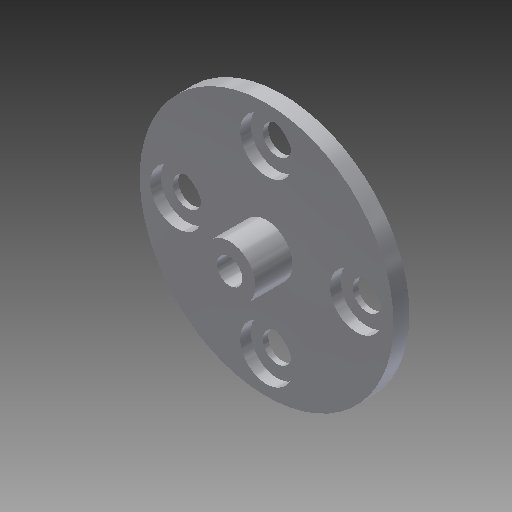
# Autodesk Inventor part: 足首_独立ピッチ_1_2
Saved by Autodesk Inventor 2018 (Build 220112000, 112)
## iProperties
Created: 2016-05-04
Part Number: 足首_独立ピッチ_1_2
Material: アルミニウム 2014-T4
Document SubType Name: Modeling
Designer: hiroaki
Density: 2.8 g/cm^3
Appearance: サテン
Mass: 1.76953 g
Surface Area: 11.344 cm^2
Volume: 0.631975 cm^3
Author: hiroaki
Autodesk Inventor part; units mm, degrees
ref_plane "YZ Plane" through (0, 0, 0) normal (1, 0, 0) x (0, 1, 0)
ref_plane "XZ Plane" through (0, 0, 0) normal (0, 1, 0) x (-1, 0, 0)
ref_plane "XY Plane" through (0, 0, 0) normal (0, 0, 1) x (1, 0, 0)
sketch "スケッチ1" plane through (0, 0, 0) normal (0, 0, 1) x (1, 0, 0)
  circle A0 centre (0, 0) radius 12
  circle A1 centre (0, 8.5) radius 1.35
  circle A2 centre (0, 0) radius 1.2
  circle A3 centre (-8.5, 0) radius 1.35
  circle A4 centre (0, -8.5) radius 1.35
  circle A5 centre (8.5, 0) radius 1.35
  dimension "d0" = 2.7
  dimension "d1" = 8.5
  dimension "d2" = 24
  dimension "d3" = 2.4
  dimension "d6" = 360
  constraints: 6 centre point, 2 coincident, 1 vertical alignment, 9 other
  measures "d0" diameter of A1
  measures "d1" distance of point (0, 0) A1.centre
  measures "d2" diameter of A0
  measures "d3" diameter of A2
extrude "押し出し1" add sketch "スケッチ1" along normal blind 1.5
sketch "スケッチ2" plane through (0, 0, 1.5) normal (0, 0, 1) x (1, 0, 0)
  circle A0 centre (0, 0) radius 1.2 projected
  circle A1 centre (0, 0) radius 12 projected
  circle A2 centre (0, 0) radius 2.45
  dimension "d10" = 4.9
  constraints: 1 centre point, 1 coincident
  measures "d10" diameter of A2
extrude "押し出し2" add sketch "スケッチ2" along normal blind 3.5 contours A2
sketch "スケッチ3" plane through (0, 0, 1.5) normal (0, 0, 1) x (1, 0, 0)
  circle A0 centre (0, 0) radius 2.45 projected
  circle A1 centre (0, 8.5) radius 1.35 projected
  point P0 (-8.5, 0)
  point P1 (0, -8.5)
  point P2 (8.5, 0)
  dimension "d15" = 360
  constraints: 1 coincident, 5 other
hole "穴1" at (0, 8.5, 1.5) at (-8.5, 0, 1.5) at (0, -8.5, 1.5) at (8.5, 0, 1.5) direction (0, 0, -1) diameter 5 depth 1
